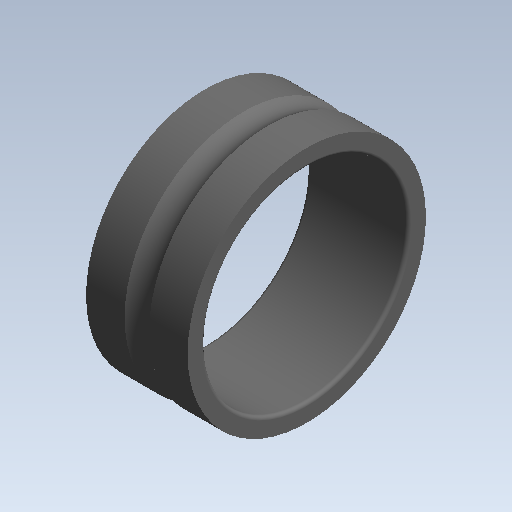
# Autodesk Inventor part: MR106ZZ1 Inner Ring
Saved by Autodesk Inventor 2021.3 (Build 253353010, 353A)
## iProperties
Part Number: MR106ZZ1 Inner Ring
Material: 一般
Catalog Web Link: www.cadenas.de
Description: shielde_type_zz_zzs_IR-
Vendor: NSK_RB
Document SubType Name: Modeling
Designer: partserver
Manufacturer: NSK_RB
Mass: 0.0305884 g
Surface Area: 1.43362 cm^2
Volume: 0.0305884 cm^3
Density: 1 g/cm^3
Appearance: PSOLRGB-128-128-128
Category: PARTsolutions
Company: NSK_RB
PSOL_IDENT_0: {$CADENAS_DATA\23d-libs\nsk_rb\roller_bearings\deep_groove_bb\exstra_small_miniatur_bb\metric_design
PSOL_IDENT_1: \shielded_type_zz_zzs_ir.prj},195 {VTYP=3D},{NB=MR106ZZ1 Inner Ring},{LINA=MR106ZZ1 Inner Ring},{NN=
PSOL_IDENT_2: shielde_type_zz_zzs_IR},{DATE=25.05.2021 06:41:25},{GEOMDATE=04.01.2008 00:00:00},{VERSION=},{LINEID=
PSOL_IDENT_3: 600},{WBVAR=},{WBNUMERIC=}  {NB=MR106ZZ1 Inner Ring},{LINA=MR106ZZ1 Inner Ring},{KT=DUMMY},{IDNR=},{
PSOL_IDENT_4: STAN=Standard},{ORDER=MR106ZZ1},{SD=6.0},{X=6.0},{DI1=7.04},{DI2=7.04},{SDE1=8.90},{SDE2=9.25},{D=10
PSOL_IDENT_5: },{DD=10},{B=0.0},{B1=3.0},{R=0.00},{R1=0.10},{CR1=495},{COR1=218},{CR2=51},{COR2=22.0},{LG=45000},{
PSOL_IDENT_6: LO=53000},{DA=0.0},{DB=7.0},{DA1=0.0},{DB1=9.3},{RA=0.00},{RB=0.10},{MASS=0.68},{SC=1},{N=16}
NB: MR106ZZ1 Inner Ring
NN: shielde_type_zz_zzs_IR
NBSYN: $ORDER. Inner Ring
LINA: MR106ZZ1 Inner Ring
CATALOG: NSK Rolling Bearing
STAN: Standard
ORDER: MR106ZZ1
SD: 6
X: 6
DI1: 7.04
DI2: 7.04
SDE1: 8.9
SDE2: 9.25
D: 10
DD: 10
B: 0
B1: 3
R: 0
R1: 0.1
CR1: 495
COR1: 218
CR2: 51
COR2: 22
LG: 45000
LO: 53000
DA: 0
DB: 7
DA1: 0
DB1: 9.3
RA: 0
RB: 0.1
MASS: 0.68
SC: 1
SUPPLIER: NSK_RB
ARTICLENO: MR106ZZ1 Inner Ring
BOMINFO: MR106ZZ1 Inner Ring
CREATOR: CADENAS GmbH
Title: MR106ZZ1 Inner Ring
Author: Cadenas PARTsolutions
Autodesk Inventor part; units mm, degrees
sketch "Sketch_1" plane through (0, 0, 0) normal (0, 0, 1) x (1, 0, 0)
  line L0 (3, 0) -> (0, 0)
  arc A0 (0, 3.1) -> (0.1, 3) centre (0.1, 3.1) ccw
  line L1 (0.1, 3) -> (2.9, 3)
  arc A1 (2.9, 3) -> (3, 3.1) centre (2.9, 3.1) ccw
  line L2 (3, 3.1) -> (3, 3.52)
  line L3 (3, 3.52) -> (1.86, 3.52)
  arc A2 (1.14, 3.52) -> (1.86, 3.52) centre (1.5, 4) ccw
  line L4 (1.14, 3.52) -> (0, 3.52)
  line L5 (0, 3.52) -> (0, 3.1)
  constraints: 12 end point, 6 point on circle, 3 centre point
revolve "Revolution1" add sketch "Sketch_1" angle 360 about axis through (3, 0, 0) along (1, 0, 0)
ref_plane "ip_st_ir_1_1_XY" through (1.5, 4, 0) normal (1, 0, 0) x (0, 0, -1)
ref_plane "ip_st_ir_1_1_YZ" through (1.5, 4, 0) normal (0, 0, -1) x (0, 1, 0)
ref_plane "ip_st_ir_1_1_ZX" through (1.5, 4, 0) normal (0, 1, 0) x (1, 0, 0)
ref_plane "ip_st_ir_1_10_XY" through (1.5, -3.6955, -1.5307) normal (1, 0, 0) x (0, 0, -1)
ref_plane "ip_st_ir_1_10_YZ" through (1.5, -3.6955, -1.5307) normal (0, 0, -1) x (0, 1, 0)
ref_plane "ip_st_ir_1_10_ZX" through (1.5, -3.6955, -1.5307) normal (0, 1, 0) x (1, 0, 0)
ref_plane "ip_st_ir_1_11_XY" through (1.5, -2.8284, -2.8284) normal (1, 0, 0) x (0, 0, -1)
ref_plane "ip_st_ir_1_11_YZ" through (1.5, -2.8284, -2.8284) normal (0, 0, -1) x (0, 1, 0)
ref_plane "ip_st_ir_1_11_ZX" through (1.5, -2.8284, -2.8284) normal (0, 1, 0) x (1, 0, 0)
ref_plane "ip_st_ir_1_12_XY" through (1.5, -1.5307, -3.6955) normal (1, 0, 0) x (0, 0, -1)
ref_plane "ip_st_ir_1_12_YZ" through (1.5, -1.5307, -3.6955) normal (0, 0, -1) x (0, 1, 0)
ref_plane "ip_st_ir_1_12_ZX" through (1.5, -1.5307, -3.6955) normal (0, 1, 0) x (1, 0, 0)
ref_plane "ip_st_ir_1_13_XY" through (1.5, 0, -4) normal (1, 0, 0) x (0, 0, -1)
ref_plane "ip_st_ir_1_13_YZ" through (1.5, 0, -4) normal (0, 0, -1) x (0, 1, 0)
ref_plane "ip_st_ir_1_13_ZX" through (1.5, 0, -4) normal (0, 1, 0) x (1, 0, 0)
ref_plane "ip_st_ir_1_14_XY" through (1.5, 1.5307, -3.6955) normal (1, 0, 0) x (0, 0, -1)
ref_plane "ip_st_ir_1_14_YZ" through (1.5, 1.5307, -3.6955) normal (0, 0, -1) x (0, 1, 0)
ref_plane "ip_st_ir_1_14_ZX" through (1.5, 1.5307, -3.6955) normal (0, 1, 0) x (1, 0, 0)
ref_plane "ip_st_ir_1_15_XY" through (1.5, 2.8284, -2.8284) normal (1, 0, 0) x (0, 0, -1)
ref_plane "ip_st_ir_1_15_YZ" through (1.5, 2.8284, -2.8284) normal (0, 0, -1) x (0, 1, 0)
ref_plane "ip_st_ir_1_15_ZX" through (1.5, 2.8284, -2.8284) normal (0, 1, 0) x (1, 0, 0)
ref_plane "ip_st_ir_1_16_XY" through (1.5, 3.6955, -1.5307) normal (1, 0, 0) x (0, 0, -1)
ref_plane "ip_st_ir_1_16_YZ" through (1.5, 3.6955, -1.5307) normal (0, 0, -1) x (0, 1, 0)
ref_plane "ip_st_ir_1_16_ZX" through (1.5, 3.6955, -1.5307) normal (0, 1, 0) x (1, 0, 0)
ref_plane "ip_st_ir_1_2_XY" through (1.5, 3.6955, 1.5307) normal (1, 0, 0) x (0, 0, -1)
ref_plane "ip_st_ir_1_2_YZ" through (1.5, 3.6955, 1.5307) normal (0, 0, -1) x (0, 1, 0)
ref_plane "ip_st_ir_1_2_ZX" through (1.5, 3.6955, 1.5307) normal (0, 1, 0) x (1, 0, 0)
ref_plane "ip_st_ir_1_3_XY" through (1.5, 2.8284, 2.8284) normal (1, 0, 0) x (0, 0, -1)
ref_plane "ip_st_ir_1_3_YZ" through (1.5, 2.8284, 2.8284) normal (0, 0, -1) x (0, 1, 0)
ref_plane "ip_st_ir_1_3_ZX" through (1.5, 2.8284, 2.8284) normal (0, 1, 0) x (1, 0, 0)
ref_plane "ip_st_ir_1_4_XY" through (1.5, 1.5307, 3.6955) normal (1, 0, 0) x (0, 0, -1)
ref_plane "ip_st_ir_1_4_YZ" through (1.5, 1.5307, 3.6955) normal (0, 0, -1) x (0, 1, 0)
ref_plane "ip_st_ir_1_4_ZX" through (1.5, 1.5307, 3.6955) normal (0, 1, 0) x (1, 0, 0)
ref_plane "ip_st_ir_1_5_XY" through (1.5, 0, 4) normal (1, 0, 0) x (0, 0, -1)
ref_plane "ip_st_ir_1_5_YZ" through (1.5, 0, 4) normal (0, 0, -1) x (0, 1, 0)
ref_plane "ip_st_ir_1_5_ZX" through (1.5, 0, 4) normal (0, 1, 0) x (1, 0, 0)
ref_plane "ip_st_ir_1_6_XY" through (1.5, -1.5307, 3.6955) normal (1, 0, 0) x (0, 0, -1)
ref_plane "ip_st_ir_1_6_YZ" through (1.5, -1.5307, 3.6955) normal (0, 0, -1) x (0, 1, 0)
ref_plane "ip_st_ir_1_6_ZX" through (1.5, -1.5307, 3.6955) normal (0, 1, 0) x (1, 0, 0)
ref_plane "ip_st_ir_1_7_XY" through (1.5, -2.8284, 2.8284) normal (1, 0, 0) x (0, 0, -1)
ref_plane "ip_st_ir_1_7_YZ" through (1.5, -2.8284, 2.8284) normal (0, 0, -1) x (0, 1, 0)
ref_plane "ip_st_ir_1_7_ZX" through (1.5, -2.8284, 2.8284) normal (0, 1, 0) x (1, 0, 0)
ref_plane "ip_st_ir_1_8_XY" through (1.5, -3.6955, 1.5307) normal (1, 0, 0) x (0, 0, -1)
ref_plane "ip_st_ir_1_8_YZ" through (1.5, -3.6955, 1.5307) normal (0, 0, -1) x (0, 1, 0)
ref_plane "ip_st_ir_1_8_ZX" through (1.5, -3.6955, 1.5307) normal (0, 1, 0) x (1, 0, 0)
ref_plane "ip_st_ir_1_9_XY" through (1.5, -4, 0) normal (1, 0, 0) x (0, 0, -1)
ref_plane "ip_st_ir_1_9_YZ" through (1.5, -4, 0) normal (0, 0, -1) x (0, 1, 0)
ref_plane "ip_st_ir_1_9_ZX" through (1.5, -4, 0) normal (0, 1, 0) x (1, 0, 0)
ref_plane "ip_st_ir_1a_XY" through (0, 0, 0) normal (1, 0, 0) x (0, 0, -1)
ref_plane "ip_st_ir_1a_YZ" through (0, 0, 0) normal (0, 0, -1) x (0, 1, 0)
ref_plane "ip_st_ir_1a_ZX" through (0, 0, 0) normal (0, 1, 0) x (1, 0, 0)
ref_plane "ip_st_ir_2a_XY" through (0.1992, 0, 0) normal (1, 0, 0) x (0, 0, -1)
ref_plane "ip_st_ir_2a_YZ" through (0.1992, 0, 0) normal (0, 0, -1) x (0, 1, 0)
ref_plane "ip_st_ir_2a_ZX" through (0.1992, 0, 0) normal (0, 1, 0) x (1, 0, 0)
body "Solid1"
